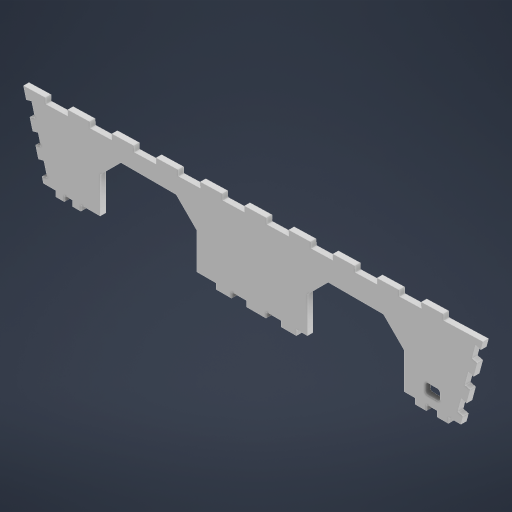
# Autodesk Inventor part: Langbektang houder
Saved by Autodesk Inventor 2023.2 (Build 272271000, 271)
## iProperties
Created: 2020-09-09
Part Number: Langbektang houder
Material: Generic
Document SubType Name: Modeling
Designer: nathan.bollaert
Density: 1 g/cm^3
Appearance: Default
Author: nathan.bollaert
Autodesk Inventor part; units mm, degrees
ref_plane "YZ Plane" through (0, 0, 0) normal (1, 0, 0) x (0, 1, 0)
ref_plane "XZ Plane" through (0, 0, 0) normal (0, 1, 0) x (-1, 0, 0)
ref_plane "XY Plane" through (0, 0, 0) normal (0, 0, 1) x (1, 0, 0)
sketch "Sketch1" plane through (0, 0, 0) normal (0, 0, 1) x (1, 0, 0)
  line L0 (0, 0) -> (300, 0)
  line L1 (300, 0) -> (318.1173, 67.6148)
  line L2 (0, 0) -> (-15.5291, 57.9555)
  line L3 (0, 0) -> (60, 0) construction
  line L4 (-15.5291, 57.9555) -> (318.1173, 67.6148)
  line L5 (8, 0) -> (14, 0)
  line L6 (14, 0) -> (14, 4)
  line L7 (8, 4) -> (8, 0)
  line L8 (20, 0) -> (26, 0)
  line L9 (26, 0) -> (26, 4)
  line L10 (20, 4) -> (20, 0)
  line L11 (135, 4) -> (135, 0)
  line L12 (135, 0) -> (124, 0)
  line L13 (124, 0) -> (124, 4)
  line L14 (160, 4) -> (160, 0)
  line L15 (160, 0) -> (146, 0)
  line L16 (146, 0) -> (146, 4)
  line L17 (8, 4) -> (-1.0718, 4)
  line L18 (14, 4) -> (20, 4)
  line L19 (40, 0) -> (40, 30)
  line L20 (110, 0) -> (110, 30)
  line L21 (182, 4) -> (182, 0)
  line L22 (182, 0) -> (171, 0)
  line L23 (171, 0) -> (171, 4)
  line L24 (26, 4) -> (40, 4)
  line L25 (124, 4) -> (110, 4)
  line L26 (146, 4) -> (135, 4)
  line L27 (160, 4) -> (171, 4)
  line L28 (190, 0) -> (190, 30)
  line L29 (182, 4) -> (190, 4)
  line L30 (95, 45) -> (110, 30)
  line L31 (55, 45) -> (40, 30)
  line L32 (55, 45) -> (95, 45)
  line L33 (260, 0) -> (260, 30)
  line L34 (260, 0) -> (290, 0) construction
  line L35 (260, 4) -> (268, 4)
  line L36 (268, 4) -> (268, 0)
  line L37 (268, 0) -> (276, 0)
  line L38 (276, 0) -> (276, 4)
  line L39 (276, 4) -> (284, 4)
  line L40 (284, 4) -> (284, 0)
  line L41 (284, 0) -> (292, 0)
  line L42 (292, 0) -> (292, 4)
  line L43 (292, 4) -> (301.0718, 4)
  line L44 (190, 30) -> (205, 45)
  line L45 (205, 45) -> (245, 45)
  line L46 (245, 45) -> (260, 30)
  line L47 (302.5882, 9.6593) -> (298.7245, 10.6945)
  line L48 (298.7245, 10.6945) -> (301.3127, 20.3538)
  line L49 (301.3127, 20.3538) -> (305.1764, 19.3185)
  line L50 (307.7646, 28.9778) -> (303.9009, 30.0131)
  line L51 (303.9009, 30.0131) -> (306.4891, 39.6723)
  line L52 (306.4891, 39.6723) -> (310.3528, 38.637)
  line L53 (309.0772, 49.3316) -> (311.6654, 58.9908)
  line L54 (312.941, 48.2963) -> (309.0772, 49.3316)
  line L55 (311.6654, 58.9908) -> (315.5291, 57.9555)
  line L56 (-2.0706, 7.7274) -> (1.7932, 8.7627)
  line L57 (1.7932, 8.7627) -> (-0.795, 18.4219)
  line L58 (-0.795, 18.4219) -> (-4.6587, 17.3867)
  line L59 (-6.7293, 25.1141) -> (-2.8656, 26.1493)
  line L60 (-2.8656, 26.1493) -> (-4.9361, 33.8768)
  line L61 (-4.9361, 33.8768) -> (-8.7998, 32.8415)
  line L62 (-10.8704, 40.5689) -> (-7.0067, 41.6042)
  line L63 (-7.0067, 41.6042) -> (-9.5949, 51.2634)
  line L64 (-9.5949, 51.2634) -> (-13.4586, 50.2281)
  line L65 (0.4642, 58.4186) -> (0.5799, 54.4202)
  line L66 (0.5799, 54.4202) -> (16.5732, 54.8833)
  line L67 (16.5732, 54.8833) -> (16.4575, 58.8816)
  line L68 (16.4575, 58.8816) -> (0.4642, 58.4186)
  line L69 (0.4642, 58.4186) -> (-15.5291, 57.9555)
  line L70 (32.4508, 59.3446) -> (32.5665, 55.3463)
  line L71 (32.5665, 55.3463) -> (48.5598, 55.8093)
  line L72 (48.5598, 55.8093) -> (48.4441, 59.8076)
  line L73 (48.4441, 59.8076) -> (32.4508, 59.3446)
  line L74 (32.4508, 59.3446) -> (16.4575, 58.8816)
  line L75 (64.4374, 60.2706) -> (64.5531, 56.2723)
  line L76 (64.5531, 56.2723) -> (80.5464, 56.7353)
  line L77 (80.5464, 56.7353) -> (80.4307, 60.7336)
  line L78 (80.4307, 60.7336) -> (64.4374, 60.2706)
  line L79 (64.4374, 60.2706) -> (48.4441, 59.8076)
  line L80 (96.424, 61.1967) -> (80.4307, 60.7336)
  line L81 (96.424, 61.1967) -> (96.5397, 57.1983)
  line L82 (112.4173, 61.6597) -> (96.424, 61.1967)
  line L83 (112.533, 57.6613) -> (112.4173, 61.6597)
  line L84 (96.5397, 57.1983) -> (112.533, 57.6613)
  line L85 (128.4105, 62.1227) -> (112.4173, 61.6597)
  line L86 (128.4105, 62.1227) -> (128.5263, 58.1244)
  line L87 (144.4038, 62.5857) -> (128.4105, 62.1227)
  line L88 (144.5196, 58.5874) -> (144.4038, 62.5857)
  line L89 (128.5263, 58.1244) -> (144.5196, 58.5874)
  line L90 (160.5129, 59.0504) -> (176.5062, 59.5134)
  line L91 (160.3971, 63.0487) -> (144.4038, 62.5857)
  line L92 (160.3971, 63.0487) -> (160.5129, 59.0504)
  line L93 (176.3904, 63.5117) -> (160.3971, 63.0487)
  line L94 (208.4928, 60.4394) -> (208.377, 64.4378)
  line L95 (192.4995, 59.9764) -> (208.4928, 60.4394)
  line L96 (208.377, 64.4378) -> (192.3837, 63.9747)
  line L97 (192.3837, 63.9747) -> (192.4995, 59.9764)
  line L98 (192.3837, 63.9747) -> (176.3904, 63.5117)
  line L99 (176.5062, 59.5134) -> (176.3904, 63.5117)
  line L100 (240.4794, 61.3655) -> (240.3636, 65.3638)
  line L101 (224.4861, 60.9025) -> (240.4794, 61.3655)
  line L102 (240.3636, 65.3638) -> (224.3703, 64.9008)
  line L103 (224.3703, 64.9008) -> (224.4861, 60.9025)
  line L104 (224.3703, 64.9008) -> (208.377, 64.4378)
  line L105 (256.3569, 65.8268) -> (240.3636, 65.3638)
  line L106 (256.3569, 65.8268) -> (256.4727, 61.8285)
  line L107 (256.4727, 61.8285) -> (272.466, 62.2915)
  line L108 (272.3502, 66.2898) -> (256.3569, 65.8268)
  line L109 (272.466, 62.2915) -> (272.3502, 66.2898)
  line L110 (288.3435, 66.7528) -> (288.4593, 62.7545)
  line L111 (304.3368, 67.2159) -> (288.3435, 66.7528)
  line L112 (288.3435, 66.7528) -> (272.3502, 66.2898)
  line L113 (317.0821, 63.7511) -> (318.1173, 67.6148)
  line L114 (317.0821, 63.7511) -> (288.4593, 62.7545)
  point P0 (3.4641, 4)
  dimension "d271" = 105
  dimension "d273" = 105
  dimension "d276" = 8
  dimension "d277" = 6
  dimension "d278" = 6
  dimension "d279" = 6
  dimension "d281" = 11
  dimension "d282" = 11
  dimension "d283" = 30
  dimension "d284" = 14
  dimension "d285" = 70
  dimension "d286" = 14
  dimension "d287" = 14
  dimension "d288" = 11
  dimension "d289" = 11
  dimension "d290" = 8
  dimension "d297" = 15
  dimension "d298" = 15
  dimension "d303" = 70
  dimension "d304" = 8
  dimension "d305" = 8
  dimension "d307" = 8
  dimension "d308" = 8
  dimension "d309" = 4
  dimension "d312" = 8
  dimension "d313" = 10
  dimension "d314" = 10
  dimension "d315" = 10
  dimension "d316" = 10
  dimension "d319" = 10
  dimension "d321" = 10
  dimension "d322" = 10
  dimension "d323" = 8
  dimension "d324" = 10
  dimension "d325" = 8
  dimension "d326" = 10
  dimension "d327" = 8
  dimension "d328" = 8
  dimension "d329" = 8
  dimension "d333" = 16
  dimension "d334" = 16
  constraints: 223 end point, 58 perpendicular, 31 parallel, 28 collinear, 22 point on line, 8 horizontal, 4 equal length, 4 vertical, 3 horizontal alignment, 1 midpoint, 43 other
  measures "d276" distance from line of L3.start L7
  measures "d277" distance of L8.end L8.start
  measures "d278" distance of L5.end L8.start
  measures "d279" distance of L5.end L5.start
  measures "d281" distance between parallel lines of L11 L13
  measures "d282" distance of L11.end L15.end
  measures "d283" distance of L19.end L19.start
  measures "d284" distance of L19.start L8.end
  measures "d285" distance of L20.start L19.start
  measures "d286" distance of L12.end L20.start
  measures "d287" distance of L14.end L15.end
  measures "d288" distance of L21.end L22.end
  measures "d289" distance of L22.end L14.end
  measures "d290" distance of L21.end L28.start
  measures "d297" distance from line of L32 L19.end
  measures "d298" horizontal distance of L31.start L19.end
  measures "d303" distance of L28.start L33.start
  measures "d304" distance of L35.start L35.end
  measures "d305" distance of L36.end L37.end
  measures "d307" distance of L38.end L39.end
  measures "d308" distance of L40.end L41.end
  measures "d312" distance of point (300, 0) L41.end
  measures "d313" distance of point (300, 0) L47.start
  measures "d314" distance of L49.end L47.start
  measures "d315" distance of L49.end L50.start
  measures "d316" distance of L52.end L50.start
  measures "d319" distance of L55.end L54.start
  measures "d321" distance of L54.start L52.end
  measures "d322" distance of L113.end L55.end
  measures "d323" distance of L3.start L56.start
  measures "d324" distance of L58.end L56.start
  measures "d325" distance of L61.end L59.start
  measures "d326" distance of L64.end L62.start
  measures "d327" distance of L59.start L58.end
  measures "d328" distance of L62.start L61.end
  measures "d329" distance of L69.end L64.end
  measures "d333" distance of L69.end L65.start
  measures "d334" distance of L65.start L67.end
extrude "Extrusion1" add sketch "Sketch1" against normal blind 4 contours L7 L17 L2 L56 L57 L58 L59 L60 L61 L62 L63 L64 L4 L65 L66 L67 L70 L71 L72 L75 L76 L77 L81 L84 L83 L86 L89 L88 L92 L90 L99 L97 L95 L94 L103 L101 L100 L106 L107 L109 L110 L114 L1 L55 L53 L54 L52 L51 L50 L49 L48 L47 L43 L42 L0 L40 L39 L38 L36 L35 L33 L46 L45 L44 L28 L29 L21 L23 L27 L14 L16 L26 L11 L13 L25 L20 L30 L32 L31 L19 L24 L9 L10 L18 L6
sketch "Sketch2" plane through (0, 0, 0) normal (0, 0, 1) x (1, 0, 0)
  line L0 (277, 18) -> (284, 18)
  line L1 (286, 16) -> (286, 12)
  line L2 (284, 10) -> (277, 10)
  line L3 (275, 12) -> (275, 16)
  arc A0 (277, 18) -> (275, 16) centre (277, 16) ccw
  arc A1 (284, 10) -> (286, 12) centre (284, 12) ccw
  arc A2 (286, 16) -> (284, 18) centre (284, 16) ccw
  arc A3 (275, 12) -> (277, 10) centre (277, 12) ccw
  line L4 (292, 4) -> (301.0718, 4) projected
  line L5 (292, 0) -> (292, 4) projected
  point P0 (0, 0)
  point P1 (286, 10)
  point P2 (286, 18)
  point P3 (275, 10)
  dimension "d339" = 11
  dimension "d340" = 8
  dimension "d341" = 2
  dimension "d342" = 6
  dimension "d346" = 6
  constraints: 8 end point, 8 point on circle, 8 tangent, 6 point on line, 4 centre point, 3 equal radius, 2 parallel, 1 horizontal, 1 perpendicular
  measures "d339" distance of point (286, 10) point (275, 10)
  measures "d340" distance of point (286, 18) point (286, 10)
  measures "d341" radius of A0
  measures "d342" distance from line of L4 point (286, 10)
  measures "d346" distance from line of L5 point (286, 10)
extrude "Extrusion2" cut sketch "Sketch2" against normal blind 4
body "Solid6"
